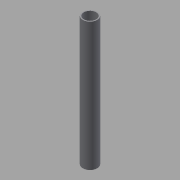
# Autodesk Inventor part: tubo corto
Saved by Autodesk Inventor 2014 (Build 180170000, 170)
## iProperties
Created: 2016-10-24
Part Number: tubo corto
Material: Steel, Alloy
Document SubType Name: Modeling
Designer: Cristian
Density: 1 g/cm^3
Appearance: Semi-Polished
Author: Cristian
Autodesk Inventor part; units mm, degrees
ref_plane "YZ Plane" through (0, 0, 0) normal (1, 0, 0) x (0, 1, 0)
ref_plane "XZ Plane" through (0, 0, 0) normal (0, 1, 0) x (-1, 0, 0)
ref_plane "XY Plane" through (0, 0, 0) normal (0, 0, 1) x (1, 0, 0)
sketch "Sketch1" plane through (0, 0, 0) normal (0, 0, 1) x (1, 0, 0)
  circle A0 centre (0, 0) radius 12
  circle A1 centre (0, 0) radius 14
  dimension "d0" = 24
  dimension "d1" = 2
  constraints: 2 centre point, 2 coincident
  measures "d0" diameter of A0
  measures "d1" radial gap between concentric circles of A1 A0
extrude "Extrusion1" add sketch "Sketch1" along normal blind 250
body "Solid1"
